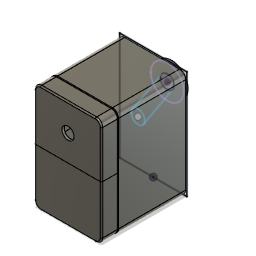
Sharpener_MUJI_Nao v4 (Autodesk Fusion 360 design; units mm, degrees)
Autodesk Fusion 360 part; units mm, degrees
note: some values were not read from the file. Set by a fixed rule: which face or edge a step refers to.
sketch "Esquisse1" plane through (0, 0, 0) normal (0, 0, 1) x (1, 0, 0)
  line L0 (27.5, 0) -> (-27.5, 0)
  line L1 (-27.5, 0) -> (-27.5, 88.5)
  line L2 (-27.5, 88.5) -> (27.5, 88.5)
  line L3 (27.5, 88.5) -> (27.5, 0)
  dimension "d1" = 55
  dimension "d2" = 88.5
  constraint horizontal L0
  constraint vertical L1
  constraint horizontal L2
  constraint vertical L3
  constraint midpoint L0 origin
  measures "d1" distance of L1.end L2.end
  measures "d2" distance of L0.end L1.end
extrude "Extrusion1" add sketch "Esquisse1" along normal blind 56 makes body 1
fillet "Congé1" radius 5 4 edges at (-27.5, 88.5, 28) (27.5, 88.5, 28) (27.5, 0, 28) (-27.5, 0, 28) on bodies 1
shell "Coque1" thickness 2 removed faces 1 at (-9.1667, 31.1667, 56) on bodies 1
sketch "Esquisse2" plane through (0, 0, 56) normal (0, 0, 1) x (1, 0, 0)
  arc A0 (-25.5, 5) -> (-22.5, 2) centre (-22.5, 5) ccw
  line L0 (-25.5, 5) -> (-25.5, 83.5)
  arc A1 (-22.5, 86.5) -> (-25.5, 83.5) centre (-22.5, 83.5) ccw
  line L1 (-22.5, 86.5) -> (22.5, 86.5)
  arc A2 (25.5, 83.5) -> (22.5, 86.5) centre (22.5, 83.5) ccw
  line L2 (25.5, 83.5) -> (25.5, 5)
  arc A3 (22.5, 2) -> (25.5, 5) centre (22.5, 5) ccw
  line L3 (22.5, 2) -> (-22.5, 2)
  arc A4 (-27.5, 5) -> (-22.5, 0) centre (-22.5, 5) ccw
  line L4 (-22.5, 0) -> (22.5, 0)
  arc A5 (22.5, 0) -> (27.5, 5) centre (22.5, 5) ccw
  line L5 (27.5, 5) -> (27.5, 83.5)
  arc A6 (27.5, 83.5) -> (22.5, 88.5) centre (22.5, 83.5) ccw
  line L6 (22.5, 88.5) -> (-22.5, 88.5)
  arc A7 (-22.5, 88.5) -> (-27.5, 83.5) centre (-22.5, 83.5) ccw
  line L7 (-27.5, 83.5) -> (-27.5, 5)
  arc A8 (-25.5, 5) -> (-22.5, 2) centre (-22.5, 5) ccw
  line L8 (-22.5, 2) -> (22.5, 2)
  arc A9 (22.5, 2) -> (25.5, 5) centre (22.5, 5) ccw
  line L9 (25.5, 5) -> (25.5, 83.5)
  arc A10 (25.5, 83.5) -> (22.5, 86.5) centre (22.5, 83.5) ccw
  line L10 (22.5, 86.5) -> (-22.5, 86.5)
  arc A11 (-22.5, 86.5) -> (-25.5, 83.5) centre (-22.5, 83.5) ccw
  line L11 (-25.5, 83.5) -> (-25.5, 5)
  line L12 (-27.5, 45) -> (27.5, 45)
  dimension "d12" = 45
  constraint coincident L7 L12.start
  constraint coincident L5 L12.end
  constraint perpendicular L5 L12
  measures "d12" distance of L4 L12
extrude "Extrusion2" add sketch "Esquisse2" along normal blind 14 separate body contours A0 L0 L2 A3 L3 A8 L8 A9 L9 L11 L12 | A0 L0 L2 A3 L3 A4 L4 A5 L5 L7 A8 L8 A9 L9 L11 L12 makes body 2
extrude "Extrusion3" add sketch "Esquisse2" against normal up to surface (54 mm away) contours A0 L0 L2 A3 L3 A8 L8 A9 L9 L11 L12 bodies 2
shell "Coque2" thickness 2 removed faces 1 at (-8.5, 45, 20) on bodies 2
fillet "Congé2" radius 1 5 edges at (-27.5, 25, 70) (-26.0355, 1.4645, 70) (0, 0, 70) (26.0355, 1.4645, 70) (27.5, 25, 70) on bodies 2
fillet "Congé3" radius 1 8 edges at (26.0355, 1.4645, 0) (0, 0, 0) (-26.0355, 1.4645, 0) (-27.5, 44.25, 0) (-26.0355, 87.0355, 0) (0, 88.5, 0) (26.0355, 87.0355, 0) (27.5, 44.25, 0) on bodies 1
fillet "Congé4" radius 2.5 5 edges at (-23.5, 25, 58) (-23.2071, 4.2929, 58) (0, 4, 58) (23.2071, 4.2929, 58) (23.5, 25, 58) on bodies 2
fillet "Congé5" radius 1 5 edges at (-27.5, 25, 56) (-26.0355, 1.4645, 56) (0, 0, 56) (26.0355, 1.4645, 56) (27.5, 25, 56) on bodies 2
extrude "Extrusion4" add sketch "Esquisse2" along normal blind 14 separate body contours L0 A1 L1 A2 L2 L5 A6 L6 A7 L7 L9 A10 L10 A11 L11 L12 | L0 A1 L1 A2 L2 L9 A10 L10 A11 L11 L12 makes body 3
extrude "Extrusion5" add sketch "Esquisse2" against normal up to surface (54 mm away) contours L0 A1 L1 A2 L2 L9 A10 L10 A11 L11 L12 bodies 3
sketch "Esquisse4" plane through (0, 0, 0) normal (0, 0, 1) x (1, 0, 0)
shell "Coque3" thickness 2 removed faces 1 at (-8.5, 45, 20) on bodies 3
extrude "Extrusion6" cut 1 faces at (7.5, 58.1667, 4) along direction (0, 0, -1) blind 10 on bodies 3 bodies 3
fillet "Congé6" radius 2.5 5 edges at (23.5, 64.25, 58) (23.2071, 84.2071, 58) (0, 84.5, 58) (-23.2071, 84.2071, 58) (-23.5, 64.25, 58) on bodies 3
fillet "Congé7" radius 1 10 edges at (27.5, 64.25, 56) (26.0355, 87.0355, 56) (0, 88.5, 56) (-26.0355, 87.0355, 56) (-27.5, 64.25, 56) (27.5, 64.25, 70) (26.0355, 87.0355, 70) (0, 88.5, 70) (-26.0355, 87.0355, 70) (-27.5, 64.25, 70) on bodies 3
hole "Perçage1" at (0, 66.1877, 70) direction (0, 0, -1) diameter 10 depth 20 tip angle 118 bodies 3
sketch "Esquisse5" plane through (0, 0, 0) normal (0, 0, 1) x (1, 0, 0)
  circle A0 centre (0, 62) radius 17.5
  dimension "d36" = 35
  measures "d36" diameter of A0
extrude "Extrusion7" add sketch "Esquisse5" against normal blind 8 bodies 1
sketch "Esquisse6" plane through (0, 0, -8) normal (0, 0, -1) x (-1, 0, 0)
  circle A0 centre (0, 62) radius 17.5
  circle A1 centre (0, 62) radius 13.5
  dimension "d39" = 27
  constraint concentric A0 A1
  measures "d39" diameter of A1
extrude "Extrusion8" add sketch "Esquisse6" along normal blind 7 contours A1 bodies 1
ref_plane "Plan de construction1" through (0, 62, -11.5) normal (0, 0, -1) x (-1, 0, 0)
sketch "Esquisse7" plane through (0, 0, -11.5) normal (0, 0, -1) x (-1, 0, 0)
  circle A0 centre (0, 62) radius 5.5
  circle A1 centre (24.0039, 25.1244) radius 5.5
  line L0 (-4.6095, 58.9995) -> (19.3944, 22.1239)
  line L1 (4.6095, 65.0005) -> (28.6134, 28.1248)
  circle A2 centre (0, 62) radius 13.5
  dimension "d43" = 11
  dimension "d44" = 44
  constraint coincident A0 L0.start
  constraint coincident A1 L0.end
  constraint tangent A1 L0
  constraint coincident A0 L1.start
  constraint coincident A1 L1.end
  constraint tangent A1 L1
  constraint tangent A0 L1
  constraint tangent A0 L0
  constraint parallel L0 L1
  constraint concentric A0 A2
  measures "d43" diameter of A0
  measures "d44" distance of L0.start L0.end
extrude "Extrusion9" add sketch "Esquisse7" along normal mid plane 4 separate body contours A0 | A0 L0 L1 A2 | A1 L0 L1 A2 | A1 picked at (2.5453, 51.4955) makes body 4
extrude "Extrusion10" add sketch "Esquisse7" along normal blind 19 separate body contours A1 makes body 5
equation "d44 = 49.5 mm - 5.5 mm"
